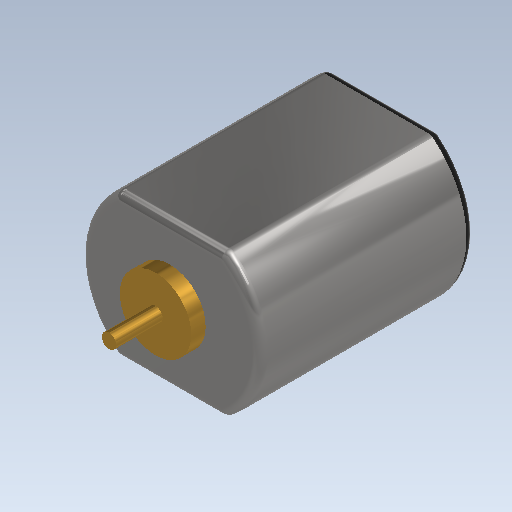
# Autodesk Inventor part: Моторчик
Saved by Autodesk Inventor 2020 (Build 240168000, 168)
## iProperties
Created: 2018-08-24
Part Number: Моторчик
Material: Латунь, мягкая, желтая
Document SubType Name: Modeling
Designer: Shepelev
Density: 8.47 g/cm^3
Appearance: Латунь - сатинированная
Author: Shepelev
Autodesk Inventor part; units mm, degrees
ref_plane "YZ Plane" through (0, 0, 0) normal (1, 0, 0) x (0, 1, 0)
ref_plane "XZ Plane" through (0, 0, 0) normal (0, 1, 0) x (-1, 0, 0)
ref_plane "XY Plane" through (0, 0, 0) normal (0, 0, 1) x (1, 0, 0)
sketch "Эскиз1" plane through (0, 0, 0) normal (1, 0, 0) x (0, 1, 0)
  line L0 (0.4, 16.4596) -> (0.4, 13.8596)
  line L1 (0.4, 13.8596) -> (2, 13.8596)
  line L2 (2, 13.8596) -> (2, 13.0596)
  line L3 (2, 13.0596) -> (5, 13.0596)
  line L4 (5, 13.0596) -> (5, 1)
  line L5 (5, 1) -> (2, 1)
  line L6 (2, 1) -> (2, 0)
  line L7 (2, 0) -> (0, 0)
  line L8 (0, 0) -> (0, 16.5)
  line L9 (0, -3.302) -> (0, 19.8121) projected
  arc A0 (0.4, 16.4596) -> (0, 16.5) centre (0, 14.5) ccw
  dimension "d0" = 16.5
  dimension "d1" = 0.8
  dimension "d2" = 2.6
  dimension "d3" = 0.8
  dimension "d4" = 10
  dimension "d5" = 4
  dimension "d6" = 1
  dimension "d7" = 4
  dimension "d13" = 2
  constraints: 18 end point, 8 perpendicular, 2 point on circle, 1 centre point, 1 point on line
  measures "d0" distance of L7.end L8.end
  measures "d1" diameter of L0 L9
  measures "d2" distance of L0.start L0.end
  measures "d3" distance of L1.end L2.end
  measures "d4" diameter of L4 L9
  measures "d5" diameter of L6 L9
  measures "d6" distance between parallel lines of L7 L5
  measures "d7" diameter of L2 L9
  measures "d13" radius of A0
revolve "Вращение1" add sketch "Эскиз1" angle 360 about axis through (0, 0, -10) along (0, 0, 1)
sketch "Эскиз2" plane through (0, 0, 1) normal (0, 0, -1) x (-1, 0, 0)
  circle A0 centre (0, 0) radius 5 projected
  line L0 (-3, 4) -> (3, 4)
  line L1 (3, -4) -> (-3, -4)
  line L2 (7, 0) -> (-7, 0) projected
  dimension "d9" = 8
  constraints: 4 end point, 4 point on circle, 1 horizontal, 1 parallel, 1 other
  measures "d9" distance between parallel lines of L1 L0
extrude "Выдавливание1" cut sketch "Эскиз2" against normal blind 13.25 contours L0 A0 | A0 L1
fillet "Сопряжение1" radius 0.5 12 edges at (0, 4, 13.0596) (5, 0, 13.0596) (-5, 0, 13.0596) (0, -4, 13.0596) (3, -4, 7.0298) (-3, -4, 7.0298) (-3, 4, 7.0298) (3, 4, 7.0298) (0, -4, 1) (5, 0, 1) (-5, 0, 1) (0, 4, 1)
